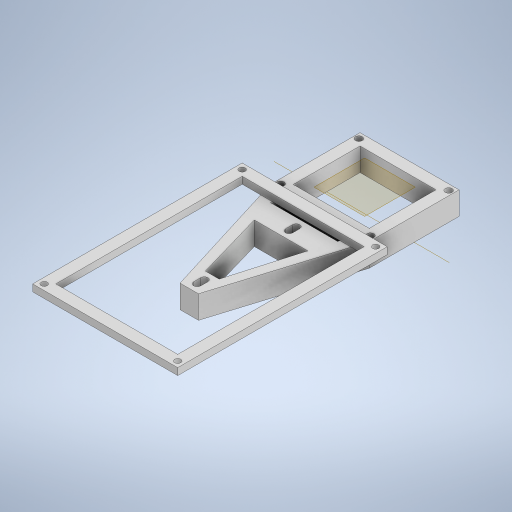
# Autodesk Inventor part: Houder Jetson Nano
Saved by Autodesk Inventor 2023.2 (Build 272271030, 271C)
## iProperties
Created: 2023-03-06
Part Number: Houder Jetson Nano
Material: Generic
Document SubType Name: Modeling
Designer: daanj
Density: 1 g/cm^3
Appearance: Default
Author: daanj
Autodesk Inventor part; units mm, degrees
ref_plane "YZ Plane" through (0, 0, 0) normal (1, 0, 0) x (0, 1, 0)
ref_plane "XZ Plane" through (0, 0, 0) normal (0, 1, 0) x (-1, 0, 0)
ref_plane "XY Plane" through (0, 0, 0) normal (0, 0, 1) x (1, 0, 0)
sketch "Sketch1" plane through (0, 0, 0) normal (0, 1, 0) x (-1, 0, 0)
  circle A0 centre (-19.5, 17) radius 1.5
  circle A1 centre (19.5, 17) radius 1.5
  circle A2 centre (-19.5, -17) radius 1.5
  circle A3 centre (19.5, -17) radius 1.5
  line L0 (16.5, 14.5) -> (16.5, -14.5)
  line L1 (-16.5, -14.5) -> (-16.5, 14.5)
  line L2 (-21.5, -19.5) -> (-21.5, 19.5)
  line L3 (-16.5, 19.5) -> (16.5, 19.5)
  line L4 (21.5, 19.5) -> (21.5, -19.5)
  line L5 (21.5, -19.5) -> (-21.5, -19.5)
  line L6 (-0.3654, -14.5) -> (-16.5, -14.5)
  line L7 (0, 0) -> (0, 19.5) construction
  line L8 (-16.5, 14.5) -> (16.5, 14.5)
  line L9 (16.5, -14.5) -> (-0.3654, -14.5)
  line L10 (21.5, 19.5) -> (4, 76.2)
  line L11 (4, 76.2) -> (-4, 76.2)
  line L12 (-4, 76.2) -> (-21.5, 19.5)
  line L13 (3, 66.2) -> (-3, 66.2)
  line L14 (11.6435, 36.3) -> (-11.6435, 36.3)
  line L15 (0, -96.6477) -> (0, 118.4334) construction
  line L16 (0, 32.85) -> (0, 29.75) construction
  line L17 (1.55, 32.85) -> (1.55, 29.75)
  line L18 (-1.55, 29.75) -> (-1.55, 32.85)
  arc A4 (1.55, 32.85) -> (-1.55, 32.85) centre (0, 32.85) ccw
  arc A5 (-1.55, 29.75) -> (1.55, 29.75) centre (0, 29.75) ccw
  line L19 (0, 72.75) -> (0, 69.65) construction
  line L20 (1.55, 72.75) -> (1.55, 69.65)
  line L21 (-1.55, 69.65) -> (-1.55, 72.75)
  arc A6 (1.55, 72.75) -> (-1.55, 72.75) centre (0, 72.75) ccw
  arc A7 (-1.55, 69.65) -> (1.55, 69.65) centre (0, 69.65) ccw
  line L22 (63.7, 0) -> (-63.7, 0) projected
  line L23 (14.5343, 26.3) -> (-14.5343, 26.3)
  line L24 (16.5, 19.5) -> (14.5343, 26.3)
  line L25 (11.6435, 36.3) -> (3, 66.2)
  line L26 (-3, 66.2) -> (-11.6435, 36.3)
  line L27 (-14.5343, 26.3) -> (-16.5, 19.5)
  point P0 (0, 31.3)
  point P1 (0, 71.2)
  dimension "d0" = 3
  dimension "d1" = 3
  dimension "d4" = 3
  dimension "d5" = 3
  dimension "d8" = 39
  dimension "d18" = 5
  dimension "d19" = 5
  dimension "d20" = 5
  dimension "d21" = 39
  dimension "d22" = 43
  dimension "d23" = 19.5
  dimension "d24" = 21.5
  dimension "d25" = 3
  dimension "d26" = 2.5
  dimension "d27" = 2.5
  dimension "d28" = 3
  dimension "d29" = 2.5
  dimension "d30" = 3
  dimension "d62" = 34
  dimension "d64" = 6
  dimension "d65" = 3
  dimension "d66" = 5
  dimension "d67" = 5
  dimension "d70" = 14.3
  dimension "d71" = 8
  dimension "d72" = 4
  dimension "d73" = 5
  dimension "d76" = 39.9
  dimension "d77" = 5
  dimension "d78" = 5
  dimension "d79" = 5
  constraints: 58 end point, 9 parallel, 8 centre point, 8 point on circle, 8 tangent, 4 point on line, 2 horizontal, 2 midpoint, 1 horizontal alignment, 1 perpendicular, 1 vertical
  measures "d0" diameter of A0
  measures "d1" diameter of A1
  measures "d4" diameter of A2
  measures "d5" diameter of A3
  measures "d8" distance of A2.centre A3.centre
  measures "d18" distance between parallel lines of L2 L1
  measures "d19" distance between parallel lines of L5 L6
  measures "d20" distance between parallel lines of L4 L0
  measures "d21" distance between parallel lines of L3 L5
  measures "d22" distance of L4.end L2.start
  measures "d23" distance from line of L3 point (0, 0)
  measures "d24" distance from line of point (0, 0) L2
  measures "d25" distance from line of L1 A0.centre
  measures "d26" distance from line of A0.centre L8
  measures "d27" distance from line of L6 A2.centre
  measures "d28" distance from line of L0 A3.centre
  measures "d29" distance from line of L6 A3.centre
  measures "d30" distance from line of L0 A1.centre
  measures "d62" distance of A1.centre A3.centre
  measures "d64" distance of L13.start L13.end
  measures "d65" distance from line of L15 L13.start
  measures "d66" distance of L3.end L4.start
  measures "d67" distance of L3.start L2.end
  measures "d70" vertical distance of A0.centre point (0, 31.3)
  measures "d71" distance of L10.end L11.end
  measures "d72" horizontal distance of L11.end point (0, 71.2)
  measures "d73" distance from line of L11 point (0, 71.2)
  measures "d76" distance of point (0, 71.2) point (0, 31.3)
  measures "d77" distance from line of L14 point (0, 31.3)
  measures "d78" distance from line of L23 point (0, 31.3)
  measures "d79" distance from line of L13 point (0, 71.2)
ref_plane "Work Plane1" through (0, 10, 0) normal (0, 1, 0) x (1, 0, 0)
extrude "Extrusion2" add sketch "Sketch1" along normal blind 10 contours L8 L1 L22 L2 L12 L11 L10 L4 L0 | L22 L4 L5 L2 L1 L6 L9 L0
sketch "Sketch2" plane through (0, 10, 0) normal (0, 1, 0) x (1, 0, 0)
  circle A0 centre (-30.2005, -23) radius 1.35
  circle A1 centre (-30.2005, -109) radius 1.35
  circle A2 centre (27.7995, -109) radius 1.35
  circle A3 centre (27.7995, -23) radius 1.35
  line L0 (-32.7005, -111.5) -> (30.2995, -111.5)
  line L1 (30.2995, -111.5) -> (30.2995, -20.5)
  line L2 (30.2995, -20.5) -> (-32.7005, -20.5)
  line L3 (-32.7005, -20.5) -> (-32.7005, -111.5)
  line L4 (-27.7005, -106.5) -> (25.2995, -106.5)
  line L5 (25.2995, -106.5) -> (25.2995, -25.5)
  line L6 (25.2995, -25.5) -> (-27.7005, -25.5)
  line L7 (-27.7005, -25.5) -> (-27.7005, -106.5)
  line L8 (-63.7, 0) -> (63.7, 0) projected
  circle A4 centre (19.5, 17) radius 1.5 projected
  point P0 (0, 0)
  dimension "d36" = 2.7
  dimension "d43" = 5
  dimension "d44" = 5
  dimension "d45" = 5
  dimension "d46" = 5
  dimension "d49" = 2.5
  dimension "d50" = 2.5
  dimension "d52" = 2.5
  dimension "d53" = 2.5
  dimension "d83" = 40
  dimension "d84" = 25.2995
  dimension "d86" = 86
  dimension "d87" = 58
  constraints: 16 end point, 5 parallel, 4 centre point, 3 equal radius, 2 horizontal alignment, 2 perpendicular, 2 vertical alignment
  measures "d36" diameter of A1
  measures "d43" distance between parallel lines of L2 L6
  measures "d44" distance between parallel lines of L3 L7
  measures "d45" distance between parallel lines of L1 L5
  measures "d46" distance between parallel lines of L0 L4
  measures "d49" distance from line of L6 A3.centre
  measures "d50" distance from line of L5 A3.centre
  measures "d52" distance from line of A2.centre L4
  measures "d53" distance from line of L7 A1.centre
  measures "d83" vertical distance of A3.centre A4.centre
  measures "d84" distance from line of point (0, 0) L5
  measures "d86" distance of A1.centre A0.centre
  measures "d87" distance of A2.centre A1.centre
extrude "Extrusion3" add sketch "Sketch2" along normal blind 3 contours L3 L2 L1 L0
equation "\"d1\" = d0"
equation "\"d4\" = d0"
equation "\"d5\" = d0"
body "Solid2"
